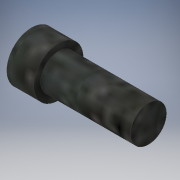
# Autodesk Inventor part: Parts_Bolt_M4_L25
Saved by Autodesk Inventor 2019.1 (Build 231200000, 200)
## iProperties
Created: 2018-08-27
Part Number: Parts_Bolt_M4_L25
Material: 鋼
Document SubType Name: Modeling
Designer: sktom
Density: 7.85 g/cm^3
Appearance: プレート
Author: sktom
Autodesk Inventor part; units mm, degrees
ref_plane "YZ Plane" through (0, 0, 0) normal (1, 0, 0) x (0, 1, 0)
ref_plane "XZ Plane" through (0, 0, 0) normal (0, 1, 0) x (-1, 0, 0)
ref_plane "XY Plane" through (0, 0, 0) normal (0, 0, 1) x (1, 0, 0)
sketch "スケッチ1" plane through (0, 0, 0) normal (0, 0, 1) x (1, 0, 0)
  line L0 (0, 0) -> (0, 2.75)
  line L1 (0, 2.75) -> (3, 2.75)
  line L2 (3, 2.75) -> (3, 2)
  line L3 (3, 2) -> (13, 2)
  line L4 (13, 2) -> (13, 0)
  line L5 (13, 0) -> (0, 0)
  dimension "d0" = 10
  dimension "d1" = 2
  dimension "d2" = 2.75
  dimension "d3" = 3
  constraints: 12 end point, 5 perpendicular, 1 vertical
  measures "d0" distance of L2.end L3.end
  measures "d1" distance of L3.end L4.end
  measures "d2" distance of L0.start L0.end
  measures "d3" distance of L0.end L1.end
revolve "回転1" add sketch "スケッチ1" angle 360 about axis through (13, 0, 0) along (-1, 0, 0)
